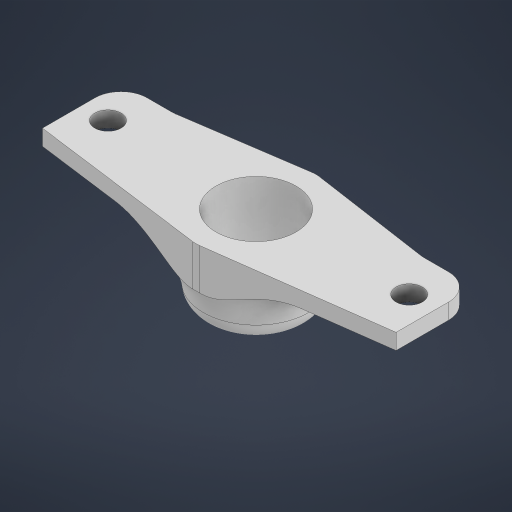
# Autodesk Inventor part: FanMotorMount
Saved by Autodesk Inventor 2023 (Build 270158000, 158)
## iProperties
Created: 2022-04-01
Part Number: FanMotorMount
Material: 一般
Document SubType Name: Modeling
Designer: neko2
Density: 1 g/cm^3
Appearance: 既定
Author: neko2
Autodesk Inventor part; units mm, degrees
ref_plane "YZ Plane" through (0, 0, 0) normal (1, 0, 0) x (0, 1, 0)
ref_plane "XZ Plane" through (0, 0, 0) normal (0, 1, 0) x (-1, 0, 0)
ref_plane "XY Plane" through (0, 0, 0) normal (0, 0, 1) x (1, 0, 0)
sketch "スケッチ7" plane through (0, 0, 0) normal (0, 1, 0) x (-1, 0, 0)
  line L0 (0, -9.199) -> (0, 0)
  line L1 (-13.5, -1.7948) -> (-13.5, -7.7948)
  line L2 (-13.5, -7.7948) -> (-9.5, -7.7948)
  circle A0 centre (0, -4.5995) radius 3.05
  line L3 (0, 0) -> (-13.5, -1.7948)
  line L4 (-9.5, -7.7948) -> (0, -9.199)
  circle A1 centre (0, -4.5948) radius 4.5547
  line L5 (13.5, -1.7948) -> (13.5, -7.7948)
  line L6 (13.5, -7.7948) -> (9.5, -7.7948)
  line L7 (0, 0) -> (13.5, -1.7948)
  line L8 (9.5, -7.7948) -> (0, -9.199)
  circle A2 centre (-11.5, -4.7948) radius 1
  circle A3 centre (11.5, -4.7948) radius 1
  point P0 (-13.5, -4.7948)
  point P1 (0.6003, -0.0798)
  point P2 (0, -0.0401)
  point P3 (0, -1.5495)
  point P4 (0, -7.6495)
  point P5 (0, -9.1495)
  point P6 (0.666, -9.1005)
  point P7 (-11.5, -7.7948)
  dimension "d38" = 6
  dimension "d39" = 4
  dimension "d40" = 27
  dimension "d41" = 6.1
  dimension "d46" = 1.5
  dimension "d55" = 2
  dimension "d61" = 0.2
  constraints: 19 end point, 4 centre point, 4 symmetric about line, 3 midpoint, 2 tangent, 2 vertical, 1 horizontal alignment, 1 perpendicular, 1 point on line, 1 vertical alignment, 1 other
  measures "d38" distance of L1.start L1.end
  measures "d39" distance of L1.end L2.end
  measures "d40" diameter of L1 L0
  measures "d41" diameter of A0
  measures "d55" diameter of A2
  measures "d61" vertical distance of A2.centre A1.centre
extrude "押し出し5" add sketch "スケッチ7" along normal blind 1.2 contours L4 A1 L0 | L0 A1 L8 | A1 L0 A0 | L0 A0 A1 | L4 L2 L1 L3 A1 | A1 L7 L5 L6 L8 | L3 L0 A1 | L7 A1 L0
fillet "フィレット6" radius 2 6 edges at (13.5, 0.6, -7.7948) (0, 0.6, 0) (9.5, 0.6, -7.7948) (-13.5, 0.6, -7.7948) (-9.5, 0.6, -7.7948) (0, 0.6, -9.199)
sketch "スケッチ10" plane through (0, 0, 0) normal (0, 1, 0) x (1, 0, 0)
  circle A0 centre (0, 4.5995) radius 3.05 projected
  circle A1 centre (0, 4.5995) radius 4
  point P0 (0, 0)
  dimension "d51" = 8
  constraints: 1 centre point, 1 coincident
  measures "d51" diameter of A1
extrude "押し出し7" add sketch "スケッチ10" against normal blind 4.5
fillet "フィレット8" radius 4 1 edges at (-4, 0, -4.5995)
sketch "スケッチ12" plane through (0, -4.5, -4.5995) normal (0, -1, 0) x (1, 0, 0)
  circle A0 centre (0, 0) radius 4 projected
  circle A1 centre (0, 0) radius 2.55
  circle A2 centre (0, 0) radius 3.05 projected
  point P0 (0, 4.5995)
  dimension "d62" = 0.5
  constraints: 1 centre point, 1 coincident
  measures "d62" radial gap between concentric circles of A1 A2
extrude "押し出し8" add sketch "スケッチ12" along normal blind 0.5 contours A0 | A2
fillet "フィレット9" radius 1.5 1 edges at (-4, -5, -4.5995)
